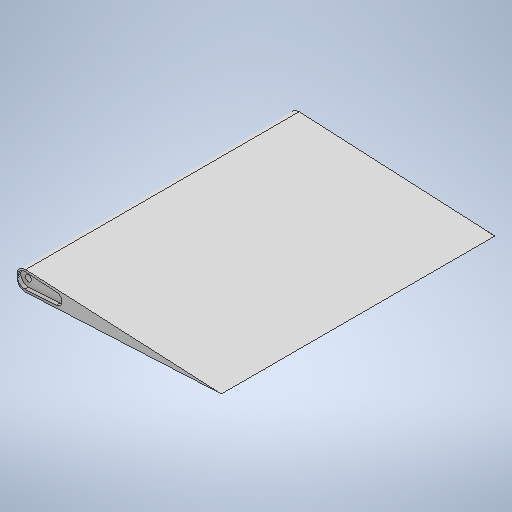
# Autodesk Inventor part: ElevatorV2
Saved by Autodesk Inventor 2025.2 (Build 292293000, 293)
## iProperties
Created: 2025-04-21
Part Number: ElevatorV2
Material: Generic
Document SubType Name: Modeling
Designer: georg
Density: 1 g/cm^3
Appearance: Default
Author: georg
Autodesk Inventor part; units mm, degrees
ref_plane "YZ Plane" through (0, 0, 0) normal (1, 0, 0) x (0, 1, 0)
ref_plane "XZ Plane" through (0, 0, 0) normal (0, 1, 0) x (-1, 0, 0)
ref_plane "XY Plane" through (0, 0, 0) normal (0, 0, 1) x (1, 0, 0)
sketch "Sketch1" plane through (0, 0, 0) normal (0, 0, 1) x (1, 0, 0)
  line L0 (357.0794, 41.0884) -> (357.0794, 43.1077)
  line L1 (362.4131, 48.1813) -> (484.0794, 42.098)
  line L2 (484.0794, 42.098) -> (362.4131, 36.0147)
  arc A0 (362.4131, 48.1813) -> (357.0794, 43.1077) centre (362.1594, 43.1077) ccw
  arc A1 (357.0794, 41.0884) -> (362.4131, 36.0147) centre (362.1594, 41.0884) ccw
  point P0 (357.0794, 35.748)
  point P1 (357.0794, 48.448)
  dimension "d0" = 127
  dimension "d1" = 12.7
  dimension "d2" = 5.08
  constraints: 6 end point, 4 point on circle, 4 point on line, 4 tangent, 2 centre point, 1 equal radius, 1 vertical
  measures "d0" distance from line of L1.end L0
  measures "d1" distance of point (357.079, 48.448) point (357.079, 35.748)
  measures "d2" radius of A0
extrude "Extrusion1" add sketch "Sketch1" along normal blind 170.0022
sketch "Sketch2" plane through (0, 0, 170.0022) normal (0, 0, 1) x (1, 0, 0)
  arc A0 (362.1294, 46.8881) -> (362.4259, 37.4357) centre (361.8271, 42.1478) ccw
  arc A1 (381.5771, 38.6478) -> (381.5771, 45.6478) centre (381.5771, 42.1478) ccw
  arc A2 (381.5771, 38.6478) -> (381.5771, 45.6478) centre (381.5771, 42.1478) ccw
  line L0 (361.8271, 37.3978) -> (381.5771, 38.6478)
  line L1 (381.5771, 45.6478) -> (362.1294, 46.8881)
  point P0 (0, 0)
  point P1 (367.7181, 34.9628)
  point P2 (367.4202, 34.9628)
  point P3 (357.0794, 41.9988)
  point P4 (356.8779, 76.4339)
  point P5 (354.6232, 35.4991)
  point P6 (354.3254, 35.4991)
  constraints: 9 point on circle, 4 end point, 3 centre point, 1 coincident, 1 point on line, 1 tangent
extrude "Extrusion2" cut sketch "Sketch2" against normal blind 2.25 contours L1 A1 L0 A0
sketch "Sketch3" plane through (0, 0, 167.7522) normal (0, 0, 1) x (1, 0, 0)
  line L0 (357.0794, 41.9988) -> (357.0794, 42.2967) projected
  arc A0 (357.0794, 41.9988) -> (361.8271, 37.3978) centre (361.8271, 42.1478) ccw projected
  line L1 (381.5771, 38.6478) -> (361.8271, 37.3978) projected
  arc A1 (381.5771, 38.6478) -> (381.5771, 45.6478) centre (381.5771, 42.1478) ccw projected
  line L2 (362.1294, 46.8881) -> (381.5771, 45.6478) projected
  arc A2 (362.1294, 46.8881) -> (357.0794, 42.2967) centre (361.8271, 42.1478) ccw projected
  circle A3 centre (361.8271, 42.1478) radius 1.905
  point P0 (0, 0)
  dimension "d7" = 3.81
  constraints: 1 centre point, 1 coincident
  measures "d7" diameter of A3
extrude "Extrusion3" cut sketch "Sketch3" against normal blind 170.18 contours A3
body "Solid1"
